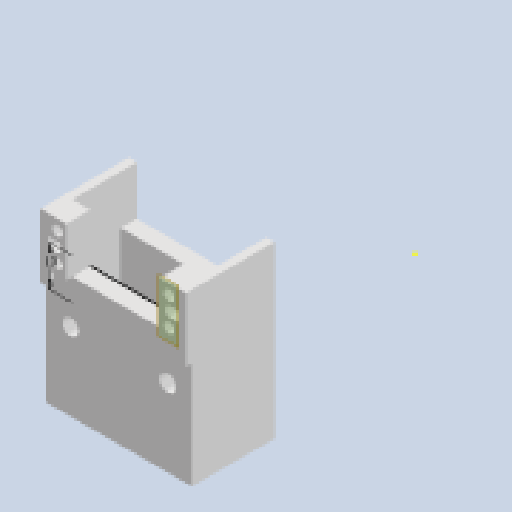
# Autodesk Inventor part: держатель сервомоторчика
Saved by Autodesk Inventor 2024.2 (Build 282272000, 272)
## iProperties
Created: 2025-11-28
Part Number: держатель сервомоторчика
Material: Типовые
Document SubType Name: Modeling
Designer: katya_notebook
Density: 1 g/cm^3
Appearance: По умолчанию
Author: katya_notebook
Autodesk Inventor part; units mm, degrees
ref_plane "YZ Plane" through (0, 0, 0) normal (1, 0, 0) x (0, 1, 0)
ref_plane "XZ Plane" through (0, 0, 0) normal (0, 1, 0) x (-1, 0, 0)
ref_plane "XY Plane" through (0, 0, 0) normal (0, 0, 1) x (1, 0, 0)
ref_plane "РабПлоскость1" through (0, 34.8975, 74.4992) normal (0, 0, -1) x (1, 0, 0)
sketch "Эскиз1" plane through (0, 34.8975, 74.4992) normal (0, 0, -1) x (1, 0, 0)
  line L0 (11.5, 6) -> (11.5, -6) projected
  line L1 (15, -6) -> (11.5, -6) projected
  arc A0 (15, -6) -> (16, -5) centre (15, -5) ccw projected
  line L2 (16, -1.25) -> (16, -5) projected
  line L3 (14, -1.25) -> (16, -1.25) projected
  arc A1 (12.8, -0.05) -> (14, -1.25) centre (14, -0.05) ccw projected
  line L4 (12.8, 0.05) -> (12.8, -0.05) projected
  arc A2 (14, 1.25) -> (12.8, 0.05) centre (14, 0.05) ccw projected
  line L5 (16, 1.25) -> (14, 1.25) projected
  line L6 (16, 5) -> (16, 1.25) projected
  arc A3 (16, 5) -> (15, 6) centre (15, 5) ccw projected
  line L7 (11.5, 6) -> (15, 6) projected
  circle A4 centre (13.75, 3.5) radius 1.25 projected
  circle A5 centre (13.75, -3.5) radius 1.25 projected
  line L8 (-11.5, -6) -> (-11.5, 6) projected
  line L9 (-15, 6) -> (-11.5, 6) projected
  arc A6 (-15, 6) -> (-16, 5) centre (-15, 5) ccw projected
  line L10 (-16, 1.3872) -> (-16, 5) projected
  line L11 (-14, 1.3872) -> (-16, 1.3872) projected
  arc A7 (-12.802, 0.1186) -> (-14, 1.3872) centre (-14, 0.1872) ccw projected
  line L12 (-12.802, 0.0186) -> (-12.802, 0.1186) projected
  arc A8 (-14, -1.25) -> (-12.802, 0.0186) centre (-14, -0.05) ccw projected
  line L13 (-16, -1.25) -> (-14, -1.25) projected
  line L14 (-16, -5) -> (-16, -1.25) projected
  arc A9 (-16, -5) -> (-15, -6) centre (-15, -5) ccw projected
  line L15 (-11.5, -6) -> (-15, -6) projected
  circle A10 centre (-13.75, 3.5) radius 1.25 projected
  circle A11 centre (-13.75, -3.5) radius 1.25 projected
  line L16 (16, 5) -> (16, 6)
  line L17 (16, 6) -> (15, 6)
  line L18 (-16, 5) -> (-16, 6)
  line L19 (-16, 6) -> (-15, 6)
  point P0 (0, 34.8975)
  constraints: 8 end point, 2 perpendicular, 2 point on line, 1 point on circle, 1 vertical
extrude "Выдавливание1" add sketch "Эскиз1" along normal blind 6
sketch "Эскиз2" plane through (0, 34.8975, 68.4992) normal (0, 0, -1) x (-1, 0, 0)
  point P0 (0, -34.8975)
sketch "Эскиз3" plane through (11.5, 28.8975, 74.4992) normal (0, -1, 0) x (1, 0, 0)
  line L0 (4.5, 0) -> (4.5, -6) projected
  line L1 (4.5, -6) -> (0, -6)
  line L2 (0, -6) -> (0, 0)
  line L3 (0, 0) -> (4.5, 0)
  line L4 (4.5, 0) -> (4.5, -6)
  line L5 (-27.5, 0) -> (-27.5, -6) projected
  line L6 (-23, 0) -> (-23, -6) projected
  line L7 (-27.5, -6) -> (-23, -6)
  line L8 (-23, -6) -> (-23, 0)
  line L9 (-23, 0) -> (-27.5, 0)
  line L10 (-27.5, 0) -> (-27.5, -6)
  line L11 (0, -6) -> (-23, -6)
  line L12 (-23, -6) -> (-23, 0)
  line L13 (-23, 0) -> (0, 0)
  line L14 (0, 0) -> (0, -6)
  line L15 (18.5784, -1.45) -> (-41.4216, -1.45) projected
  point P0 (-11.5, -74.4992)
  point P1 (4.5, -1.45)
  point P2 (-27.5, -1.45)
  constraints: 24 end point, 6 parallel, 3 horizontal, 3 perpendicular
extrude "Выдавливание2" add sketch "Эскиз3" along normal blind 30 contours L0 L1 L2 L15 | L2 L11 L6 L15 | L6 L7 L5 L15
sketch "Эскиз4" plane through (0, 34.8975, 68.4992) normal (0, 0, -1) x (-1, 0, 0)
  line L0 (-16, -6) -> (-11.5, -6) projected
  line L1 (16, -6) -> (16, -36) projected
  line L2 (-16, -6) -> (16, -6)
  line L3 (16, -6) -> (16, -16)
  line L4 (16, -16) -> (-16, -16)
  line L5 (-16, -16) -> (-16, -6)
  point P0 (16, -6)
  point P1 (-11.5, -6)
  dimension "d4" = 10
  constraints: 8 end point, 2 parallel, 1 horizontal, 1 perpendicular, 1 point on line
  measures "d4" distance of L1.start L3.end
ref_plane "РабПлоскость2" through (-11.5, 28.8975, 52.6492) normal (0, 0, -1) x (0, 1, 0)
sketch "Эскиз5" plane through (0, 34.8975, 68.4992) normal (0, 0, -1) x (-1, 0, 0)
  line L0 (-16, -36) -> (16, -36) projected
  line L1 (16, -36) -> (-16, -36)
  line L2 (-16, -36) -> (-16, -32)
  line L3 (-16, -32) -> (16, -32)
  line L4 (16, -32) -> (16, -36)
  point P0 (0, -34.8975)
  point P1 (-16, -36)
  dimension "d7" = 4
  constraints: 8 end point, 2 parallel, 1 horizontal, 1 perpendicular
  measures "d7" distance of L3.end L0.end
ref_plane "РабПлоскость3" through (-11.5, 28.8975, 52.6492) normal (0, 0, -1) x (0, 1, 0)
extrude "Выдавливание4" add sketch "Эскиз5" along normal up to surface (15.85 mm away)
sketch "Эскиз6" plane through (-16, 2.8975, 68.4992) normal (0, 1, 0) x (1, 0, 0)
  line L0 (32, -4.55) -> (32, 15.85) projected
  line L1 (0, -4.55) -> (0, 15.85) projected
  line L2 (32, 15.85) -> (0, 15.85)
  line L3 (0, 15.85) -> (0, 11.85)
  line L4 (0, 11.85) -> (32, 11.85)
  line L5 (32, 11.85) -> (32, 15.85)
  point P0 (16, 68.4992)
  point P1 (32, 11.85)
  dimension "d10" = 4
  constraints: 8 end point, 2 parallel, 1 horizontal, 1 perpendicular, 1 point on line
  measures "d10" distance of L0.end L4.end
ref_plane "РабПлоскость4" through (-15, 28.8975, 52.6492) normal (0, -1, 0) x (1, 0, 0)
extrude "Выдавливание5" add sketch "Эскиз6" along normal up to surface (26 mm away)
sketch "Эскиз7" plane through (-16, 2.8975, 68.4992) normal (0, 1, 0) x (1, 0, 0)
  line L0 (32, 11.85) -> (0, 11.85) projected
  line L1 (0, 0) -> (0, 11.85) projected
  line L2 (32, 0) -> (0, 0) projected
  line L3 (32, 0) -> (32, 11.85) projected
  point P0 (16, 68.4992)
sketch "Эскиз8" plane through (-16, 2.8975, 68.4992) normal (0, 1, 0) x (1, 0, 0)
  circle A0 centre (8, 5.925) radius 2
  circle A1 centre (24, 5.925) radius 2
  line L0 (27.5, 0) -> (31, 0) projected
  line L1 (4.5, 0) -> (27.5, 0) projected
  line L2 (0, 0) -> (0, 11.85) projected
  line L3 (32, 0) -> (32, 11.85) projected
  point P0 (16, 68.4992)
  dimension "d13" = 4
  dimension "d14" = 4
  dimension "d15" = 5.925
  dimension "d16" = 5.925
  dimension "d17" = 8
  dimension "d18" = 8
  constraints: 2 centre point
  measures "d13" diameter of A0
  measures "d14" diameter of A1
  measures "d15" distance from line of L0 A1.centre
  measures "d16" distance from line of L1 A0.centre
  measures "d17" distance from line of L2 A0.centre
  measures "d18" distance from line of L3 A1.centre
extrude "Выдавливание6" cut sketch "Эскиз8" against normal blind 10
sketch "Эскиз9" plane through (0, 34.8975, 68.4992) normal (0, 0, -1) x (-1, 0, 0)
  circle A0 centre (-12, -16.8489) radius 2
  circle A1 centre (12, -16.8489) radius 2
  line L0 (-16, -36) -> (-16, -6) projected
  line L1 (-16, -6) -> (16, -6) projected
  line L2 (16, -1.3872) -> (16, -32) projected
  point P0 (0, -34.8975)
  dimension "d21" = 4
  dimension "d22" = 4
  dimension "d24" = 4
  dimension "d25" = 24
  constraints: 2 centre point
  measures "d21" diameter of A1
  measures "d22" diameter of A0
  measures "d24" distance from line of L2 A1.centre
  measures "d25" distance of A1.centre A0.centre
extrude "Выдавливание7" cut sketch "Эскиз9" against normal blind 10
sketch "Эскиз10" plane through (16, 28.8975, 74.4992) normal (1, 0, 0) x (0, 0, -1)
  line L0 (21.85, -30) -> (21.85, 0) projected
  line L1 (21.85, -30) -> (0, -30)
  line L2 (0, -30) -> (0, 12)
  line L3 (0, 12) -> (21.85, 12)
  line L4 (21.85, 12) -> (21.85, -30)
  point P0 (74.4992, -28.8975)
  point P1 (21.85, 0)
  constraints: 8 end point, 2 parallel, 1 horizontal, 1 perpendicular
extrude "Выдавливание8" add sketch "Эскиз10" along normal blind 2
sketch "Эскиз11" plane through (16, 28.8975, 74.4992) normal (-1, 0, 0) x (0, 0, 1)
  line L0 (-6, 12) -> (-6, 0) projected
  line L1 (0, 12) -> (-6, 12)
  line L2 (-6, 12) -> (-6, 8)
  line L3 (-6, 8) -> (0, 8)
  line L4 (0, 8) -> (0, 12)
  point P0 (-74.4992, -28.8975)
  dimension "d30" = 4
  constraints: 8 end point, 2 parallel, 1 horizontal, 1 perpendicular, 1 point on line
  measures "d30" distance of L0.start L2.end
extrude "Выдавливание9" add sketch "Эскиз11" along normal blind 1
sketch "Эскиз12" plane through (-16, 36.1475, 74.4992) normal (-1, 0, 0) x (0, 0, 1)
  line L0 (-6, 4.75) -> (-6, -7.25) projected
  line L1 (0, -7.25) -> (0, 4.75) projected
  line L2 (-6, 4.75) -> (0, 4.75)
  line L3 (0, 4.75) -> (0, 0.75)
  line L4 (0, 0.75) -> (-6, 0.75)
  line L5 (-6, 0.75) -> (-6, 4.75)
  point P0 (-74.4992, -36.1475)
  point P1 (-6, 0.75)
  dimension "d33" = 4
  constraints: 8 end point, 2 parallel, 1 horizontal, 1 perpendicular, 1 point on line
  measures "d33" distance of L1.end L3.end
extrude "Выдавливание10" add sketch "Эскиз12" against normal blind 1
sketch "Эскиз13" plane through (-16, 28.8975, 74.4992) normal (-1, 0, 0) x (0, 0, 1)
  line L0 (0, 12) -> (-6, 12) projected
  line L1 (-21.85, 0) -> (-21.85, -30) projected
  line L2 (0, 12) -> (-21.85, 12)
  line L3 (-21.85, 12) -> (-21.85, -30)
  line L4 (-21.85, -30) -> (0, -30)
  line L5 (0, -30) -> (0, 12)
  point P0 (-74.4992, -28.8975)
  constraints: 8 end point, 2 parallel, 1 horizontal, 1 perpendicular
extrude "Выдавливание11" add sketch "Эскиз13" along normal blind 2
sketch "Эскиз14" plane through (11.5, -1.1025, 74.4992) normal (0, -1, 0) x (1, 0, 0)
  circle A0 centre (-3.5, -11.925) radius 2 projected
  circle A1 centre (-19.5, -11.925) radius 2 projected
  circle A2 centre (-3.5, -11.925) radius 1.5
  circle A3 centre (-19.5, -11.925) radius 1.5
  point P0 (-11.5, -74.4992)
  dimension "d38" = 3
  dimension "d39" = 3
  constraints: 2 centre point, 2 coincident
  measures "d38" diameter of A2
  measures "d39" diameter of A3
extrude "Выдавливание12" add sketch "Эскиз14" against normal blind 4
sketch "Эскиз15" plane through (18, 28.8975, 74.4992) normal (1, 0, 0) x (0, 0, -1)
  line L0 (1.45, -3.75) -> (1.45, -63.75) projected
  line L1 (-2.55, -3.75) -> (1.45, -3.75) projected
  line L2 (-2.55, -3.75) -> (1.45, -3.75)
  line L3 (1.45, -3.75) -> (1.45, -34.5952)
  line L4 (1.45, -34.5952) -> (-2.55, -34.5952)
  line L5 (-2.55, -34.5952) -> (-2.55, -3.75)
  point P0 (74.4992, -28.8975)
  constraints: 8 end point, 2 perpendicular, 1 horizontal, 1 point on line
extrude "Выдавливание13" cut sketch "Эскиз15" against normal blind 100
